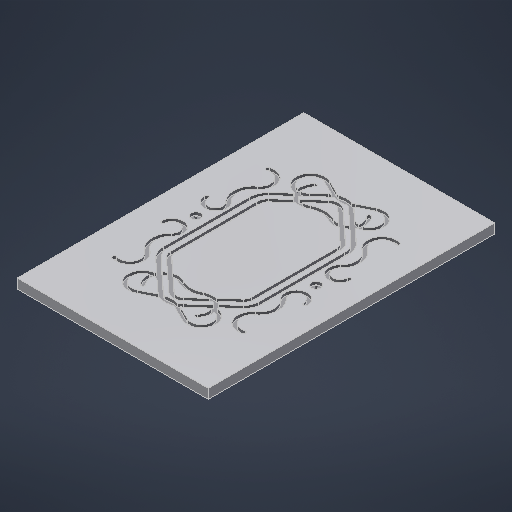
# Autodesk Inventor part: Logo Valhalla
Saved by Autodesk Inventor 2026 (Build 300175000, 175)
## iProperties
Created: 2025-06-24
Part Number: Logo Valhalla
Material: Generic
Document SubType Name: Modeling
Designer: feder
Density: 1 g/cm^3
Appearance: Default
Author: feder
Autodesk Inventor part; units mm, degrees
ref_plane "YZ Plane" through (0, 0, 0) normal (1, 0, 0) x (0, 1, 0)
ref_plane "XZ Plane" through (0, 0, 0) normal (0, 1, 0) x (-1, 0, 0)
ref_plane "XY Plane" through (0, 0, 0) normal (0, 0, 1) x (1, 0, 0)
sketch "Sketch2" plane through (0, 0, 0) normal (0, 1, 0) x (-1, 0, 0)
  arc A0 (37.5871, -50.511) -> (40, -45) centre (32.5, -45) ccw
  line L0 (40, -45) -> (40, 0)
  arc A1 (-5.0871, -80.511) -> (5.0871, -80.511) centre (0, -75) ccw
  line L1 (37.5871, -50.511) -> (5.0871, -80.511)
  line L2 (-40, 0) -> (-40, -45)
  arc A2 (-40, -45) -> (-37.5871, -50.511) centre (-32.5, -45) ccw
  line L3 (-5.0871, -80.511) -> (-37.5871, -50.511)
  arc A3 (40, 45) -> (37.5871, 50.511) centre (32.5, 45) ccw
  line L4 (40, 0) -> (40, 45)
  arc A4 (-37.5871, 50.511) -> (-40, 45) centre (-32.5, 45) ccw
  line L5 (-40, 0) -> (-40, 45)
  arc A5 (5.0871, 80.511) -> (-5.0871, 80.511) centre (0, 75) ccw
  line L6 (37.5871, 50.511) -> (5.0871, 80.511)
  line L7 (-5.0871, 80.511) -> (-37.5871, 50.511)
  line L8 (44, -45) -> (44, 45)
  arc A6 (40.3002, -53.4502) -> (44, -45) centre (32.5, -45) ccw
  line L9 (40.3002, -53.4502) -> (7.8002, -83.4502)
  arc A7 (-7.8002, -83.4502) -> (7.8002, -83.4502) centre (0, -75) ccw
  arc A8 (7.8002, 83.4502) -> (-7.8002, 83.4502) centre (0, 75) ccw
  arc A9 (44, 45) -> (40.3002, 53.4502) centre (32.5, 45) ccw
  arc A10 (-40.3002, 53.4502) -> (-44, 45) centre (-32.5, 45) ccw
  arc A11 (-44, -45) -> (-40.3002, -53.4502) centre (-32.5, -45) ccw
  line L10 (-7.8002, -83.4502) -> (-40.3002, -53.4502)
  line L11 (-44, -45) -> (-44, 45)
  line L12 (-40.3002, 53.4502) -> (-7.8002, 83.4502)
  line L13 (40.3002, 53.4502) -> (7.8002, 83.4502)
  arc A12 (-10.5133, -86.3895) -> (10.5133, -86.3895) centre (0, -75) ccw
  arc A13 (-13.2265, -89.3287) -> (13.2265, -89.3287) centre (0, -75) ccw
  arc A14 (-52, -45) -> (-45.7265, -59.3287) centre (-32.5, -45) ccw
  arc A15 (-48, -45) -> (-43.0133, -56.3895) centre (-32.5, -45) ccw
  line L14 (52, 0) -> (52, -45)
  line L15 (13.2265, -89.3287) -> (45.7265, -59.3287)
  line L16 (10.5133, -86.3895) -> (43.0133, -56.3895)
  line L17 (48, 0) -> (48, -45)
  arc A16 (43.0133, -56.3895) -> (48, -45) centre (32.5, -45) ccw
  arc A17 (45.7265, -59.3287) -> (52, -45) centre (32.5, -45) ccw
  line L18 (-10.5133, -86.3895) -> (-43.0133, -56.3895)
  line L19 (-13.2265, -89.3287) -> (-45.7265, -59.3287)
  line L20 (-52, 0) -> (-52, -45)
  line L21 (-48, 0) -> (-48, -45)
  line L22 (-48, 0) -> (-52, 0)
  line L23 (52, 0) -> (48, 0)
  point P0 (0, 0)
  dimension "d13" = 7.5
  dimension "d14" = 32.5
  dimension "d15" = 45
  dimension "d16" = 40
  dimension "d17" = 7.5
  dimension "d18" = 75
  dimension "d19" = 40
  dimension "d20" = 7.5
  dimension "d21" = 32.5
  dimension "d22" = 7.5
  dimension "d23" = 45
  dimension "d24" = 32.5
  dimension "d25" = 7.5
  dimension "d26" = 32.5
  dimension "d27" = 45
  dimension "d28" = 7.5
  dimension "d29" = 75
  dimension "d54" = 44
  dimension "d55" = 11.5
  dimension "d57" = 11.5
  dimension "d58" = 11.5
  dimension "d59" = 11.5
  dimension "d60" = 11.5
  dimension "d61" = 11.5
  dimension "d62" = 44
  dimension "d65" = 15.5
  dimension "d66" = 19.5
  dimension "d71" = 15.5
  dimension "d72" = 19.5
  dimension "d74" = 52
  dimension "d75" = 48
  dimension "d76" = 19.5
  dimension "d77" = 15.5
  dimension "d78" = 52
  dimension "d79" = 48
  constraints: 48 end point, 36 point on circle, 25 tangent, 18 centre point, 12 coincident, 10 vertical, 2 equal length, 2 horizontal alignment, 2 vertical alignment, 1 horizontal
  measures "d13" radius of A0
  measures "d14" horizontal distance of point (0, 0) A0.centre
  measures "d15" vertical distance of point (0, 0) A0.centre
  measures "d16" distance of point (0, 0) L0.end
  measures "d17" radius of A1
  measures "d18" distance of point (0, 0) A1.centre
  measures "d19" distance of point (0, 0) L2.start
  measures "d20" radius of A2
  measures "d21" horizontal distance of point (0, 0) A2.centre
  measures "d22" radius of A3
  measures "d23" vertical distance of point (0, 0) A3.centre
  measures "d24" horizontal distance of point (0, 0) A3.centre
  measures "d25" radius of A4
  measures "d26" horizontal distance of point (0, 0) A4.centre
  measures "d27" vertical distance of point (0, 0) A4.centre
  measures "d28" radius of A5
  measures "d29" distance of A5.centre point (0, 0)
  measures "d54" distance from line of point (0, 0) L8
  measures "d55" radius of A6
  measures "d57" radius of A7
  measures "d58" radius of A8
  measures "d59" radius of A9
  measures "d60" radius of A10
  measures "d61" radius of A11
  measures "d62" distance from line of point (0, 0) L11
  measures "d65" radius of A12
  measures "d66" radius of A13
  measures "d71" radius of A15
  measures "d72" radius of A14
  measures "d74" distance from line of L14 point (0, 0)
  measures "d75" distance from line of point (0, 0) L17
  measures "d76" radius of A17
  measures "d77" radius of A16
  measures "d78" distance from line of point (0, 0) L20
  measures "d79" distance of point (0, 0) L21.start
sketch "Sketch4" plane through (0, 0, 0) normal (0, 1, 0) x (-1, 0, 0)
  line L0 (100, -150) -> (-100, -150)
  line L1 (-100, -150) -> (-100, 150)
  line L2 (-100, 150) -> (100, 150)
  line L3 (100, 150) -> (100, -150)
  point P0 (0, 0)
  point P1 (100, 0)
  point P2 (0, -150)
  dimension "d45" = 200
  dimension "d46" = 300
  constraints: 8 end point, 2 midpoint, 2 parallel, 1 horizontal, 1 horizontal alignment, 1 perpendicular, 1 vertical alignment
  measures "d45" distance of L0.start L0.end
  measures "d46" distance of L0.end L1.end
extrude "Extrusion1" add sketch "Sketch4" against normal blind 10
extrude "Extrusion4" cut sketch "Sketch2" against normal blind 3.5
mirror "Mirror1" about plane through (0, 0, 0) normal (0, 0, 1) of "Extrusion4"
sketch "Sketch6" plane through (0, 0, 0) normal (0, 1, 0) x (-1, 0, 0)
  arc A0 (-40, -45) -> (-37.5871, -50.511) centre (-32.5, -45) ccw projected
  line L0 (-37.5871, -50.511) -> (-5.0871, -80.511) projected
  arc A1 (-5.0871, -80.511) -> (5.0871, -80.511) centre (0, -75) ccw projected
  line L1 (5.0871, -80.511) -> (37.5871, -50.511) projected
  arc A2 (37.5871, -50.511) -> (40, -45) centre (32.5, -45) ccw projected
  line L2 (40, -45) -> (40, 45) projected
  arc A3 (40, 45) -> (37.5871, 50.511) centre (32.5, 45) ccw projected
  line L3 (37.5871, 50.511) -> (5.0871, 80.511) projected
  arc A4 (5.0871, 80.511) -> (-5.0871, 80.511) centre (0, 75) ccw projected
  line L4 (-5.0871, 80.511) -> (-37.5871, 50.511) projected
  arc A5 (-37.5871, 50.511) -> (-40, 45) centre (-32.5, 45) ccw projected
  line L5 (-40, 45) -> (-40, -45) projected
  arc A6 (-13.2265, -89.3287) -> (13.2265, -89.3287) centre (0, -75) ccw projected
  line L6 (-43.0133, -56.3895) -> (-10.5133, -86.3895) projected
  arc A7 (-10.5133, -86.3895) -> (10.5133, -86.3895) centre (0, -75) ccw projected
  line L7 (-13.2265, -89.3287) -> (-45.7265, -59.3287) projected
  arc A8 (11.5541, -90.7083) -> (-11.5541, -90.7083) centre (0, -114) ccw
  arc A9 (9.7573, -94.2821) -> (-9.7571, -94.282) centre (0, -114) ccw
  arc A10 (-20.7091, -76.9779) -> (-24.2308, -101.4441) centre (-30.8833, -88) ccw
  circle A11 centre (-30.8833, -88) radius 11
  line L8 (-9.7571, -94.282) -> (-24.2308, -101.4441)
  line L9 (-11.5312, -90.6969) -> (-26.0048, -97.859)
  circle A12 centre (30.883, -88) radius 11
  arc A13 (24.2303, -101.444) -> (15.9283, -86.8346) centre (30.883, -88) ccw
  line L10 (10.5133, -86.3895) -> (43.0133, -56.3895) projected
  line L11 (45.7265, -59.3287) -> (13.2265, -89.3287) projected
  line L12 (24.2303, -101.444) -> (9.7573, -94.2821)
  line L13 (26.0043, -97.8589) -> (11.5314, -90.697)
  arc A14 (-10.519, -65.4536) -> (0, -68) centre (0, -45) ccw
  arc A15 (-12.3484, -69.0108) -> (0, -72) centre (0, -45) ccw
  arc A16 (-12.3484, -69.0108) -> (-26.867, -88.607) centre (-18, -80) ccw
  arc A17 (-10.519, -65.4536) -> (-29.7372, -91.393) centre (-18, -80) ccw
  arc A18 (-29.7372, -91.393) -> (-26.867, -88.607) centre (-28.3021, -90) ccw
  line L14 (23.3697, -79.9657) -> (20.6478, -77.0346)
  line L15 (0, -72) -> (0, -68)
  point P0 (0, 0)
  dimension "d102" = 22
  dimension "d99" = 22
  dimension "d100" = 26
  dimension "d101" = 30
  dimension "d103" = 114
  dimension "d104" = 88
  dimension "d105" = 30.8833
  dimension "d106" = 22
  dimension "d107" = 30
  dimension "d108" = 30.883
  dimension "d109" = 23
  dimension "d110" = 27
  dimension "d111" = 45
  dimension "d112" = 18
  dimension "d113" = 80
  dimension "d115" = 2
  dimension "d116" = 90
  dimension "d117" = 28.3021
  dimension "d118" = 12.3573
  dimension "d119" = 16.3573
  constraints: 25 point on circle, 12 end point, 11 tangent, 10 centre point, 5 coincident, 4 point on line, 2 vertical alignment, 1 horizontal alignment, 1 vertical, 5 other
  measures "d99" radius of A9
  measures "d100" radius of A8
  measures "d101" diameter of A10
  measures "d103" distance of point (0, 0) A8.centre
  measures "d104" vertical distance of point (0, 0) point (-30.883, -88)
  measures "d105" horizontal distance of point (0, 0) A10.centre
  measures "d106" diameter of A12
  measures "d107" diameter of A13
  measures "d108" horizontal distance of point (0, 0) A12.centre
  measures "d109" radius of A14
  measures "d110" radius of A15
  measures "d111" distance of point (0, 0) A15.centre
  measures "d112" horizontal distance of A16.centre point (0, 0)
  measures "d113" vertical distance of point (0, 0) A16.centre
  measures "d115" radius of A18
  measures "d116" vertical distance of point (0, 0) A18.centre
  measures "d117" horizontal distance of point (0, 0) A18.centre
  measures "d118" radius of A16
  measures "d119" radius of A17
extrude "Extrusion5" cut sketch "Sketch6" against normal blind 3.5 contours A17 A14 L15 A15 A16 L0 | L0 A16 L6 A17 | L6 A16 A10 L7 A17 | L7 A10 A17 | A16 L7 A10 | L7 A16 A11 A17 A10 | A11 A16 A18 A17 picked at (-30.0627, -88.8146)
mirror "Mirror2" about plane through (0, 0, 0) normal (1, 0, 0) of "Extrusion5"
sketch "Sketch7" plane through (0, 0, 0) normal (0, 1, 0) x (1, 0, 0)
  arc A0 (-24.2303, 101.444) -> (-15.9283, 86.8346) centre (-30.883, 88) ccw projected
  arc A1 (-26.0046, 97.8588) -> (-23.4221, 79.9173) centre (-30.883, 88) ccw
  line L0 (-45.7265, 59.3287) -> (-13.2265, 89.3287) projected
  arc A2 (-24.2303, 101.444) -> (-20.7088, 76.9779) centre (-30.883, 88) ccw
  line L1 (-23.4221, 79.9173) -> (-20.7088, 76.9779)
  arc A3 (-9.7573, 94.2821) -> (9.7571, 94.282) centre (0, 114) ccw projected
  arc A4 (-9.7573, 94.2821) -> (-0.0001, 92) centre (0, 114) ccw
  line L2 (-24.2303, 101.444) -> (-9.7573, 94.2821)
  line L3 (-26.0046, 97.8588) -> (-11.531, 90.6969)
  arc A5 (-11.531, 90.6969) -> (-0.0001, 88) centre (0, 114) ccw
  circle A6 centre (0, 90) radius 2
  line L4 (-0.0001, 92) -> (-0.0001, 88)
  point P0 (0, 0)
  point P1 (-29.1359, 74.6431)
  point P2 (-9.7573, 94.2821)
  point P3 (-24.2303, 101.444)
  point P4 (-20.7088, 76.9779)
  point P5 (-0.0001, 92)
  point P6 (-0.0001, 88)
  dimension "d125" = 22
  dimension "d126" = 26
  dimension "d129" = 4
  constraints: 9 point on circle, 8 end point, 6 tangent, 5 centre point, 4 coincident, 1 concentric, 1 perpendicular, 1 point on line, 1 vertical
  measures "d125" radius of A4
  measures "d126" radius of A5
  measures "d129" diameter of A6
extrude "Extrusion6" cut sketch "Sketch7" against normal blind 3.5 contours A0 L0 L1 | A0 L2 A3 A6 A5 L3 A1 L0 | L4 A6 | A6 L4 picked at (-27.1845, 75.4575)
mirror "Mirror3" about plane through (0, 0, 0) normal (1, 0, 0) of "Extrusion6"
mirror "Mirror4" about plane through (0, 0, 0) normal (0, 0, 1) of "Extrusion6", "Mirror3", "Extrusion5", "Mirror2"
sketch "Sketch8" plane through (0, 0, 0) normal (0, 1, 0) x (1, 0, 0)
  arc A0 (68.4798, 82.3154) -> (55.4368, 55.6845) centre (64, 68) ccw
  arc A1 (67.2852, 78.498) -> (57.7534, 58.9457) centre (64, 68) ccw
  circle A2 centre (63, 0) radius 5
  circle A3 centre (63, 0) radius 1
  arc A4 (56.9057, 31.0562) -> (55.4368, 55.6845) centre (46, 42.7637) ccw
  arc A5 (59.8182, 28.3049) -> (57.4731, 59.1457) centre (46, 42.7637) ccw
  arc A6 (57.0545, 31.1966) -> (76.5, 22.8828) centre (65, 22.8828) ccw
  arc A7 (59.8182, 28.3049) -> (72.5, 22.8828) centre (65, 22.8828) ccw
  arc A8 (76.5, 22.8828) -> (72.5, 22.8828) centre (74.5, 22.8828) ccw
  arc A9 (67.2852, 78.498) -> (68.4798, 82.3154) centre (67.8825, 80.4067) ccw
  point P0 (0, 0)
  dimension "d130" = 15
  dimension "d131" = 11
  dimension "d132" = 10
  dimension "d133" = 2
  dimension "d134" = 64
  dimension "d135" = 68
  dimension "d139" = 16
  dimension "d140" = 20
  dimension "d141" = 46
  dimension "d142" = 42.7637
  dimension "d143" = 15
  dimension "d144" = 23
  dimension "d145" = 65
  dimension "d146" = 22.8828
  dimension "d147" = 2
  dimension "d149" = 4
  dimension "d150" = 2
  dimension "d151" = 63
  constraints: 19 point on circle, 10 centre point, 4 coincident, 2 tangent, 1 horizontal alignment
  measures "d130" radius of A0
  measures "d131" radius of A1
  measures "d132" diameter of A2
  measures "d133" diameter of A3
  measures "d134" horizontal distance of point (0, 0) A0.centre
  measures "d135" vertical distance of point (0, 0) A0.centre
  measures "d139" radius of A4
  measures "d140" radius of A5
  measures "d141" horizontal distance of point (0, 0) A4.centre
  measures "d142" vertical distance of point (0, 0) A4.centre
  measures "d143" diameter of A7
  measures "d144" diameter of A6
  measures "d145" horizontal distance of point (0, 0) A6.centre
  measures "d146" vertical distance of point (0, 0) A6.centre
  measures "d147" radius of A8
  measures "d149" distance of A0.start A1.start
  measures "d150" radius of A9
  measures "d151" distance of A2.centre point (0, 0)
extrude "Extrusion7" cut sketch "Sketch8" against normal blind 3.5
mirror "Mirror5" about plane through (0, 0, 0) normal (0, 0, 1) of "Extrusion7"
mirror "Mirror6" about plane through (0, 0, 0) normal (1, 0, 0) of "Extrusion7", "Mirror5"
body "Solid1"
